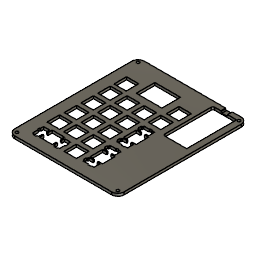
Pad+plate (Autodesk Fusion 360 design; units mm, degrees)
part number: 2026-07-29-07-50-32-719
Autodesk Fusion 360 part; units mm, degrees
(part 1 of 2)
sketch "efc796056b68a6326252bc44c872f28c73b40230_switch" plane through (0, 0, 0) normal (0, 0, 1) x (1, 0, 0)
  line L0 (-14.5057, -35.9059) -> (-14.5057, -40.6078)
  line L1 (-14.5057, -40.6078) -> (-16.0312, -40.6078)
  line L2 (-16.0312, -40.6078) -> (-16.0312, -37.3762)
  line L3 (-16.0312, -37.3762) -> (-22.7808, -37.3762)
  line L4 (-22.7808, -37.3762) -> (-22.7808, -40.6078)
  line L5 (-22.7808, -40.6078) -> (-23.6063, -40.6078)
  line L6 (-23.6063, -40.6078) -> (-23.6063, -43.4066)
  line L7 (-23.6063, -43.4066) -> (-22.7808, -43.4066)
  line L8 (-22.7808, -43.4066) -> (-22.7808, -49.6767)
  line L9 (-22.7808, -49.6767) -> (-21.0555, -49.6767)
  line L10 (-21.0555, -49.6767) -> (-21.0555, -50.8756)
  line L11 (-21.0555, -50.8756) -> (-17.7565, -50.8756)
  line L12 (-17.7565, -50.8756) -> (-17.7565, -49.6767)
  line L13 (-17.7565, -49.6767) -> (-16.0312, -49.6767)
  line L14 (-16.0312, -49.6767) -> (-16.0312, -45.2063)
  line L15 (-16.0312, -45.2063) -> (-14.5057, -45.2063)
  line L16 (-14.5057, -45.2063) -> (-14.5057, -49.9068)
  line L17 (-14.5057, -49.9068) -> (-0.5063, -49.9068)
  line L18 (-0.5063, -49.9068) -> (-0.5063, -45.2063)
  line L19 (-0.5063, -45.2063) -> (1.0192, -45.2063)
  line L20 (1.0192, -45.2063) -> (1.0192, -49.6767)
  line L21 (1.0192, -49.6767) -> (2.7445, -49.6767)
  line L22 (2.7445, -49.6767) -> (2.7445, -50.8756)
  line L23 (2.7445, -50.8756) -> (6.0436, -50.8756)
  line L24 (6.0436, -50.8756) -> (6.0436, -49.6767)
  line L25 (6.0436, -49.6767) -> (7.7689, -49.6767)
  line L26 (7.7689, -49.6767) -> (7.7689, -43.4066)
  line L27 (7.7689, -43.4066) -> (8.5943, -43.4066)
  line L28 (8.5943, -43.4066) -> (8.5943, -40.6078)
  line L29 (8.5943, -40.6078) -> (7.7689, -40.6078)
  line L30 (7.7689, -40.6078) -> (7.7689, -37.3762)
  line L31 (7.7689, -37.3762) -> (1.0192, -37.3762)
  line L32 (1.0192, -37.3762) -> (1.0192, -40.6078)
  line L33 (1.0192, -40.6078) -> (-0.5063, -40.6078)
  line L34 (-0.5063, -40.6078) -> (-0.5063, -35.9059)
  line L35 (-0.5063, -35.9059) -> (-14.5057, -35.9059)
  line L36 (14.0693, -35.9059) -> (28.0686, -35.9059)
  line L37 (28.0686, -35.9059) -> (28.0686, -49.9068)
  line L38 (28.0686, -49.9068) -> (14.0693, -49.9068)
  line L39 (14.0693, -49.9068) -> (14.0693, -35.9059)
  line L40 (39.6196, -17.2817) -> (39.6196, -18.1071)
  line L41 (39.6196, -18.1071) -> (33.3493, -18.1071)
  line L42 (33.3493, -18.1071) -> (33.3493, -19.8325)
  line L43 (33.3493, -19.8325) -> (32.1492, -19.8325)
  line L44 (32.1492, -19.8325) -> (32.1492, -23.1315)
  line L45 (32.1492, -23.1315) -> (33.3493, -23.1315)
  line L46 (33.3493, -23.1315) -> (33.3493, -24.8568)
  line L47 (33.3493, -24.8568) -> (37.8197, -24.8568)
  line L48 (37.8197, -24.8568) -> (37.8197, -26.3823)
  line L49 (37.8197, -26.3823) -> (33.1193, -26.3823)
  line L50 (33.1193, -26.3823) -> (33.1193, -40.3818)
  line L51 (33.1193, -40.3818) -> (37.8197, -40.3818)
  line L52 (37.8197, -40.3818) -> (37.8197, -41.9073)
  line L53 (37.8197, -41.9073) -> (33.3493, -41.9073)
  line L54 (33.3493, -41.9073) -> (33.3493, -43.6326)
  line L55 (33.3493, -43.6326) -> (32.1492, -43.6326)
  line L56 (32.1492, -43.6326) -> (32.1492, -46.9316)
  line L57 (32.1492, -46.9316) -> (33.3493, -46.9316)
  line L58 (33.3493, -46.9316) -> (33.3493, -48.6569)
  line L59 (33.3493, -48.6569) -> (39.6196, -48.6569)
  line L60 (39.6196, -48.6569) -> (39.6196, -49.4824)
  line L61 (39.6196, -49.4824) -> (42.4196, -49.4824)
  line L62 (42.4196, -49.4824) -> (42.4196, -48.6569)
  line L63 (42.4196, -48.6569) -> (45.6496, -48.6569)
  line L64 (45.6496, -48.6569) -> (45.6496, -41.9073)
  line L65 (45.6496, -41.9073) -> (42.4196, -41.9073)
  line L66 (42.4196, -41.9073) -> (42.4196, -40.3818)
  line L67 (42.4196, -40.3818) -> (47.1186, -40.3818)
  line L68 (47.1186, -40.3818) -> (47.1186, -26.3823)
  line L69 (47.1186, -26.3823) -> (42.4196, -26.3823)
  line L70 (42.4196, -26.3823) -> (42.4196, -24.8568)
  line L71 (42.4196, -24.8568) -> (45.6496, -24.8568)
  line L72 (45.6496, -24.8568) -> (45.6496, -18.1071)
  line L73 (45.6496, -18.1071) -> (42.4196, -18.1071)
  line L74 (42.4196, -18.1071) -> (42.4196, -17.2817)
  line L75 (42.4196, -17.2817) -> (39.6196, -17.2817)
  line L76 (-24.0307, -16.8574) -> (-10.0312, -16.8574)
  line L77 (-10.0312, -16.8574) -> (-10.0312, -30.8568)
  line L78 (-10.0312, -30.8568) -> (-24.0307, -30.8568)
  line L79 (-24.0307, -30.8568) -> (-24.0307, -16.8574)
  line L80 (-4.9807, -16.8574) -> (9.0186, -16.8574)
  line L81 (9.0186, -16.8574) -> (9.0186, -30.8568)
  line L82 (9.0186, -30.8568) -> (-4.9807, -30.8568)
  line L83 (-4.9807, -30.8568) -> (-4.9807, -16.8574)
  line L84 (14.0693, -16.8574) -> (28.0686, -16.8574)
  line L85 (28.0686, -16.8574) -> (28.0686, -30.8568)
  line L86 (28.0686, -30.8568) -> (14.0693, -30.8568)
  line L87 (14.0693, -30.8568) -> (14.0693, -16.8574)
  line L88 (-24.0307, 2.1927) -> (-10.0312, 2.1927)
  line L89 (-10.0312, 2.1927) -> (-10.0312, -11.8066)
  line L90 (-10.0312, -11.8066) -> (-24.0307, -11.8066)
  line L91 (-24.0307, -11.8066) -> (-24.0307, 2.1927)
  line L92 (-4.9807, 2.1927) -> (9.0186, 2.1927)
  line L93 (9.0186, 2.1927) -> (9.0186, -11.8066)
  line L94 (9.0186, -11.8066) -> (-4.9807, -11.8066)
  line L95 (-4.9807, -11.8066) -> (-4.9807, 2.1927)
  line L96 (14.0693, 2.1927) -> (28.0686, 2.1927)
  line L97 (28.0686, 2.1927) -> (28.0686, -11.8066)
  line L98 (28.0686, -11.8066) -> (14.0693, -11.8066)
  line L99 (14.0693, -11.8066) -> (14.0693, 2.1927)
  line L100 (39.6196, 20.8183) -> (39.6196, 19.9928)
  line L101 (39.6196, 19.9928) -> (33.3493, 19.9928)
  line L102 (33.3493, 19.9928) -> (33.3493, 18.2691)
  line L103 (33.3493, 18.2691) -> (32.1492, 18.2691)
  line L104 (32.1492, 18.2691) -> (32.1492, 14.9685)
  line L105 (32.1492, 14.9685) -> (33.3493, 14.9685)
  line L106 (33.3493, 14.9685) -> (33.3493, 13.2431)
  line L107 (33.3493, 13.2431) -> (37.8197, 13.2431)
  line L108 (37.8197, 13.2431) -> (37.8197, 11.7177)
  line L109 (37.8197, 11.7177) -> (33.1193, 11.7177)
  line L110 (33.1193, 11.7177) -> (33.1193, -2.2816)
  line L111 (33.1193, -2.2816) -> (37.8197, -2.2816)
  line L112 (37.8197, -2.2816) -> (37.8197, -3.8074)
  line L113 (37.8197, -3.8074) -> (33.3493, -3.8074)
  line L114 (33.3493, -3.8074) -> (33.3493, -5.5325)
  line L115 (33.3493, -5.5325) -> (32.1492, -5.5325)
  line L116 (32.1492, -5.5325) -> (32.1492, -8.8317)
  line L117 (32.1492, -8.8317) -> (33.3493, -8.8317)
  line L118 (33.3493, -8.8317) -> (33.3493, -10.5567)
  line L119 (33.3493, -10.5567) -> (39.6196, -10.5567)
  line L120 (39.6196, -10.5567) -> (39.6196, -11.3822)
  line L121 (39.6196, -11.3822) -> (42.4196, -11.3822)
  line L122 (42.4196, -11.3822) -> (42.4196, -10.5567)
  line L123 (42.4196, -10.5567) -> (45.6496, -10.5567)
  line L124 (45.6496, -10.5567) -> (45.6496, -3.8074)
  line L125 (45.6496, -3.8074) -> (42.4196, -3.8074)
  line L126 (42.4196, -3.8074) -> (42.4196, -2.2816)
  line L127 (42.4196, -2.2816) -> (47.1186, -2.2816)
  line L128 (47.1186, -2.2816) -> (47.1186, 11.7177)
  line L129 (47.1186, 11.7177) -> (42.4196, 11.7177)
  line L130 (42.4196, 11.7177) -> (42.4196, 13.2431)
  line L131 (42.4196, 13.2431) -> (45.6496, 13.2431)
  line L132 (45.6496, 13.2431) -> (45.6496, 19.9928)
  line L133 (45.6496, 19.9928) -> (42.4196, 19.9928)
  line L134 (42.4196, 19.9928) -> (42.4196, 20.8183)
  line L135 (42.4196, 20.8183) -> (39.6196, 20.8183)
  line L136 (-24.0307, 21.2427) -> (-10.0312, 21.2427)
  line L137 (-10.0312, 21.2427) -> (-10.0312, 7.2434)
  line L138 (-10.0312, 7.2434) -> (-24.0307, 7.2434)
  line L139 (-24.0307, 7.2434) -> (-24.0307, 21.2427)
  line L140 (-4.9807, 21.2427) -> (9.0186, 21.2427)
  line L141 (9.0186, 21.2427) -> (9.0186, 7.2434)
  line L142 (9.0186, 7.2434) -> (-4.9807, 7.2434)
  line L143 (-4.9807, 7.2434) -> (-4.9807, 21.2427)
  line L144 (14.0693, 21.2427) -> (28.0686, 21.2427)
  line L145 (28.0686, 21.2427) -> (28.0686, 7.2434)
  line L146 (28.0686, 7.2434) -> (14.0693, 7.2434)
  line L147 (14.0693, 7.2434) -> (14.0693, 21.2427)
  line L148 (-24.0307, 40.2927) -> (-10.0312, 40.2927)
  line L149 (-10.0312, 40.2927) -> (-10.0312, 26.2934)
  line L150 (-10.0312, 26.2934) -> (-24.0307, 26.2934)
  line L151 (-24.0307, 26.2934) -> (-24.0307, 40.2927)
  line L152 (-4.9807, 40.2927) -> (9.0186, 40.2927)
  line L153 (9.0186, 40.2927) -> (9.0186, 26.2934)
  line L154 (9.0186, 26.2934) -> (-4.9807, 26.2934)
  line L155 (-4.9807, 26.2934) -> (-4.9807, 40.2927)
  line L156 (14.0693, 40.2927) -> (28.0686, 40.2927)
  line L157 (28.0686, 40.2927) -> (28.0686, 26.2934)
  line L158 (28.0686, 26.2934) -> (14.0693, 26.2934)
  line L159 (14.0693, 26.2934) -> (14.0693, 40.2927)
  line L160 (33.1193, 40.2927) -> (47.1186, 40.2927)
  line L161 (47.1186, 40.2927) -> (47.1186, 26.2934)
  line L162 (47.1186, 26.2934) -> (33.1193, 26.2934)
  line L163 (33.1193, 26.2934) -> (33.1193, 40.2927)
  line L164 (-24.0307, 59.3426) -> (-10.0312, 59.3426)
  line L165 (-10.0312, 59.3426) -> (-10.0312, 45.3434)
  line L166 (-10.0312, 45.3434) -> (-24.0307, 45.3434)
  line L167 (-24.0307, 45.3434) -> (-24.0307, 59.3426)
  line L168 (33.1193, 59.3426) -> (47.1186, 59.3426)
  line L169 (47.1186, 59.3426) -> (47.1186, 45.3434)
  line L170 (47.1186, 45.3434) -> (33.1193, 45.3434)
  line L171 (33.1193, 45.3434) -> (33.1193, 59.3426)
sketch "Pad_plate _sketch" plane through (0, 0, 0) normal (0, 0, 1) x (1, 0, 0)
  line L0 (-30.0717, -55.8522) -> (79.9283, -55.8522)
  line L1 (79.9283, -55.8522) -> (79.9283, 77.1478)
  line L2 (79.9283, 77.1478) -> (-30.0717, 77.1478)
  line L3 (-30.0717, 77.1478) -> (-30.0717, -55.8522)
  circle A0 centre (74.9283, -50.8522) radius 1.5875
  circle A1 centre (-3.1217, -47.9522) radius 0.3874
  circle A2 centre (25.4533, -47.9522) radius 0.3874
  circle A3 centre (-8.2017, -43.9522) radius 1.9875
  circle A4 centre (20.3733, -43.9522) radius 1.9875
  circle A5 centre (-13.2817, -43.9522) radius 0.8624
  circle A6 centre (-3.1217, -43.9522) radius 0.8624
  circle A7 centre (15.2933, -43.9522) radius 0.8624
  circle A8 centre (25.4533, -43.9522) radius 0.8624
  circle A9 centre (-12.0117, -41.4122) radius 0.7374
  circle A10 centre (16.5633, -41.4122) radius 0.7374
  circle A11 centre (-3.1217, -40.3322) radius 0.3874
  circle A12 centre (25.4533, -40.3322) radius 0.3874
  circle A13 centre (39.4233, -39.5072) radius 0.8624
  circle A14 centre (-5.6617, -38.8722) radius 0.7374
  circle A15 centre (22.9133, -38.8722) radius 0.7374
  circle A16 centre (36.8833, -38.2372) radius 0.7374
  circle A17 centre (44.5033, -38.4272) radius 0.3874
  circle A18 centre (39.4233, -34.4272) radius 1.9875
  circle A19 centre (34.3433, -31.8872) radius 0.7374
  circle A20 centre (44.5033, -30.8072) radius 0.3874
  circle A21 centre (39.4233, -29.3472) radius 0.8624
  circle A22 centre (-12.6467, -28.9022) radius 0.3874
  circle A23 centre (6.4033, -28.9022) radius 0.3874
  circle A24 centre (25.4533, -28.9022) radius 0.3874
  circle A25 centre (-17.7267, -24.9022) radius 1.9875
  circle A26 centre (1.3233, -24.9022) radius 1.9875
  circle A27 centre (20.3733, -24.9022) radius 1.9875
  circle A28 centre (-22.8067, -24.9022) radius 0.8624
  circle A29 centre (-12.6467, -24.9022) radius 0.8624
  circle A30 centre (-3.7567, -24.9022) radius 0.8624
  circle A31 centre (6.4033, -24.9022) radius 0.8624
  circle A32 centre (15.2933, -24.9022) radius 0.8624
  circle A33 centre (25.4533, -24.9022) radius 0.8624
  circle A34 centre (-21.5367, -22.3622) radius 0.7374
  circle A35 centre (-2.4867, -22.3622) radius 0.7374
  circle A36 centre (16.5633, -22.3622) radius 0.7374
  circle A37 centre (-12.6467, -21.2822) radius 0.3874
  circle A38 centre (6.4033, -21.2822) radius 0.3874
  circle A39 centre (25.4533, -21.2822) radius 0.3874
  circle A40 centre (-15.1867, -19.8222) radius 0.7374
  circle A41 centre (3.8633, -19.8222) radius 0.7374
  circle A42 centre (22.9133, -19.8222) radius 0.7374
  circle A43 centre (-12.6467, -9.8522) radius 0.3874
  circle A44 centre (6.4033, -9.8522) radius 0.3874
  circle A45 centre (25.4533, -9.8522) radius 0.3874
  circle A46 centre (-17.7267, -5.8522) radius 1.9875
  circle A47 centre (1.3233, -5.8522) radius 1.9875
  circle A48 centre (20.3733, -5.8522) radius 1.9875
  circle A49 centre (-22.8067, -5.8522) radius 0.8624
  circle A50 centre (-12.6467, -5.8522) radius 0.8624
  circle A51 centre (-3.7567, -5.8522) radius 0.8624
  circle A52 centre (6.4033, -5.8522) radius 0.8624
  circle A53 centre (15.2933, -5.8522) radius 0.8624
  circle A54 centre (25.4533, -5.8522) radius 0.8624
  circle A55 centre (-21.5367, -3.3122) radius 0.7374
  circle A56 centre (-2.4867, -3.3122) radius 0.7374
  circle A57 centre (16.5633, -3.3122) radius 0.7374
  circle A58 centre (-12.6467, -2.2322) radius 0.3874
  circle A59 centre (6.4033, -2.2322) radius 0.3874
  circle A60 centre (25.4533, -2.2322) radius 0.3874
  circle A61 centre (39.4233, -1.4072) radius 0.8624
  circle A62 centre (-15.1867, -0.7722) radius 0.7374
  circle A63 centre (3.8633, -0.7722) radius 0.7374
  circle A64 centre (22.9133, -0.7722) radius 0.7374
  circle A65 centre (36.8833, -0.1372) radius 0.7374
  circle A66 centre (44.5033, -0.3272) radius 0.3874
  circle A67 centre (39.4233, 3.6728) radius 1.9875
  circle A68 centre (34.3433, 6.2128) radius 0.7374
  circle A69 centre (44.5033, 7.2928) radius 0.3874
  circle A70 centre (39.4233, 8.7528) radius 0.8624
  circle A71 centre (-12.6467, 9.1978) radius 0.3874
  circle A72 centre (6.4033, 9.1978) radius 0.3874
  circle A73 centre (25.4533, 9.1978) radius 0.3874
  circle A74 centre (-17.7267, 13.1978) radius 1.9875
  circle A75 centre (1.3233, 13.1978) radius 1.9875
  circle A76 centre (20.3733, 13.1978) radius 1.9875
  circle A77 centre (-22.8067, 13.1978) radius 0.8624
  circle A78 centre (-12.6467, 13.1978) radius 0.8624
  circle A79 centre (-3.7567, 13.1978) radius 0.8624
  circle A80 centre (6.4033, 13.1978) radius 0.8624
  circle A81 centre (15.2933, 13.1978) radius 0.8624
  circle A82 centre (25.4533, 13.1978) radius 0.8624
  circle A83 centre (-21.5367, 15.7378) radius 0.7374
  circle A84 centre (-2.4867, 15.7378) radius 0.7374
  circle A85 centre (16.5633, 15.7378) radius 0.7374
  circle A86 centre (-12.6467, 16.8178) radius 0.3874
  circle A87 centre (6.4033, 16.8178) radius 0.3874
  circle A88 centre (25.4533, 16.8178) radius 0.3874
  circle A89 centre (-15.1867, 18.2778) radius 0.7374
  circle A90 centre (3.8633, 18.2778) radius 0.7374
  circle A91 centre (22.9133, 18.2778) radius 0.7374
  circle A92 centre (57.1483, 27.0478) radius 0.4974
  circle A93 centre (74.9283, 27.0478) radius 0.4974
  circle A94 centre (63.4983, 27.2778) radius 0.4974
  circle A95 centre (66.0383, 27.2778) radius 0.4974
  circle A96 centre (68.5783, 27.2778) radius 0.4974
  circle A97 centre (-12.6467, 28.2478) radius 0.3874
  circle A98 centre (6.4033, 28.2478) radius 0.3874
  circle A99 centre (25.4533, 28.2478) radius 0.3874
  circle A100 centre (44.5033, 28.2478) radius 0.3874
  circle A101 centre (57.1483, 29.5878) radius 0.4974
  circle A102 centre (74.9283, 29.5878) radius 0.4974
  circle A103 centre (-17.7267, 32.2478) radius 1.9875
  circle A104 centre (1.3233, 32.2478) radius 1.9875
  circle A105 centre (20.3733, 32.2478) radius 1.9875
  circle A106 centre (39.4233, 32.2478) radius 1.9875
  circle A107 centre (-22.8067, 32.2478) radius 0.8624
  circle A108 centre (-12.6467, 32.2478) radius 0.8624
  circle A109 centre (-3.7567, 32.2478) radius 0.8624
  circle A110 centre (6.4033, 32.2478) radius 0.8624
  circle A111 centre (15.2933, 32.2478) radius 0.8624
  circle A112 centre (25.4533, 32.2478) radius 0.8624
  circle A113 centre (34.3433, 32.2478) radius 0.8624
  circle A114 centre (44.5033, 32.2478) radius 0.8624
  circle A115 centre (57.1483, 32.1278) radius 0.4974
  circle A116 centre (74.9283, 32.1278) radius 0.4974
  circle A117 centre (-8.5767, 33.7828) radius 0.3874
  circle A118 centre (-21.5367, 34.7878) radius 0.7374
  circle A119 centre (-2.4867, 34.7878) radius 0.7374
  circle A120 centre (16.5633, 34.7878) radius 0.7374
  circle A121 centre (35.6133, 34.7878) radius 0.7374
  circle A122 centre (57.1483, 34.6678) radius 0.4974
  circle A123 centre (74.9283, 34.6678) radius 0.4974
  circle A124 centre (29.4233, 35.7828) radius 0.3874
  circle A125 centre (-12.6467, 35.8678) radius 0.3874
  circle A126 centre (6.4033, 35.8678) radius 0.3874
  circle A127 centre (25.4533, 35.8678) radius 0.3874
  circle A128 centre (44.5033, 35.8678) radius 0.3874
  circle A129 centre (-15.1867, 37.3278) radius 0.7374
  circle A130 centre (3.8633, 37.3278) radius 0.7374
  circle A131 centre (22.9133, 37.3278) radius 0.7374
  circle A132 centre (41.9633, 37.3278) radius 0.7374
  circle A133 centre (57.1483, 37.2078) radius 0.4974
  circle A134 centre (74.9283, 37.2078) radius 0.4974
  circle A135 centre (57.1483, 39.7478) radius 0.4974
  circle A136 centre (74.9283, 39.7478) radius 0.4974
  circle A137 centre (-8.5767, 41.4028) radius 0.3874
  circle A138 centre (57.1483, 42.2878) radius 0.4974
  circle A139 centre (74.9283, 42.2878) radius 0.4974
  circle A140 centre (29.4233, 43.4028) radius 0.3874
  line L4 (-17.927, 45.7303) -> (-19.2264, 45.7303)
  line L5 (-19.9324, 44.7787) -> (-19.8771, 44.6451)
  arc A141 (-19.2264, 45.7303) -> (-19.9324, 44.7787) centre (-19.2266, 44.9928) ccw
  arc A142 (-17.927, 44.2553) -> (-17.927, 45.7303) centre (-17.9268, 44.9928) ccw
  arc A143 (-19.8771, 44.6451) -> (-19.2264, 44.2553) centre (-19.2265, 44.9929) ccw
  line L6 (-19.2264, 44.2553) -> (-17.927, 44.2553)
  circle A144 centre (57.1483, 44.8278) radius 0.4974
  circle A145 centre (74.9283, 44.8278) radius 0.4974
  line L7 (41.073, 46.2303) -> (39.7736, 46.2303)
  arc A146 (39.7736, 46.2303) -> (39.0676, 45.2787) centre (39.7734, 45.4928) ccw
  arc A147 (39.1229, 45.1451) -> (39.7736, 44.7553) centre (39.7735, 45.4929) ccw
  line L8 (39.0676, 45.2787) -> (39.1229, 45.1451)
  arc A148 (41.073, 44.7553) -> (41.073, 46.2303) centre (41.0732, 45.4928) ccw
  line L9 (39.7736, 44.7553) -> (41.073, 44.7553)
  circle A149 centre (57.1483, 47.3678) radius 0.4974
  circle A150 centre (74.9283, 47.3678) radius 0.4974
  circle A151 centre (-26.0767, 48.0928) radius 0.4874
  circle A152 centre (-11.5767, 48.0928) radius 0.4874
  circle A153 centre (32.9233, 48.5928) radius 0.4874
  circle A154 centre (47.4233, 48.5928) radius 0.4874
  circle A155 centre (0.4238, 49.6478) radius 1.0875
  circle A156 centre (7.1183, 49.1478) radius 0.4874
  circle A157 centre (9.6583, 49.1478) radius 0.4874
  circle A158 centre (12.1983, 49.1478) radius 0.4874
  circle A159 centre (14.7383, 49.1478) radius 0.4874
  circle A160 centre (57.1483, 49.9078) radius 0.4974
  circle A161 centre (74.9283, 49.9078) radius 0.4974
  circle A162 centre (-18.5767, 50.5928) radius 1.0374
  line L10 (-23.3764, 49.8053) -> (-22.777, 49.8053)
  line L11 (-24.1302, 50.3642) -> (-24.0712, 50.2216)
  arc A163 (-22.777, 49.8053) -> (-22.777, 51.3803) centre (-22.7768, 50.5928) ccw
  arc A164 (-23.3764, 51.3803) -> (-24.1302, 50.3642) centre (-23.3766, 50.5928) ccw
  line L12 (-22.777, 51.3803) -> (-23.3764, 51.3803)
  arc A165 (-24.0712, 50.2216) -> (-23.3764, 49.8053) centre (-23.3765, 50.5929) ccw
  circle A166 centre (40.4233, 51.0928) radius 1.0374
  circle A167 centre (-26.0767, 50.5928) radius 0.4874
  line L13 (34.8698, 50.8642) -> (34.9288, 50.7216)
  arc A168 (35.6236, 51.8803) -> (34.8698, 50.8642) centre (35.6234, 51.0928) ccw
  line L14 (35.6236, 50.3053) -> (36.223, 50.3053)
  line L15 (36.223, 51.8803) -> (35.6236, 51.8803)
  arc A169 (34.9288, 50.7216) -> (35.6236, 50.3053) centre (35.6235, 51.0929) ccw
  arc A170 (36.223, 50.3053) -> (36.223, 51.8803) centre (36.2232, 51.0928) ccw
  circle A171 centre (32.9233, 51.0928) radius 0.4874
  circle A172 centre (57.1483, 52.4478) radius 0.4974
  circle A173 centre (74.9283, 52.4478) radius 0.4974
  circle A174 centre (-26.0767, 53.0928) radius 0.4874
  circle A175 centre (-11.5767, 53.0928) radius 0.4874
  circle A176 centre (32.9233, 53.5928) radius 0.4874
  circle A177 centre (47.4233, 53.5928) radius 0.4874
  circle A178 centre (57.1483, 54.9878) radius 0.4974
  circle A179 centre (74.9283, 54.9878) radius 0.4974
  arc A180 (-19.2264, 56.9303) -> (-19.9324, 55.9787) centre (-19.2266, 56.1928) ccw
  arc A181 (-17.927, 55.4553) -> (-17.927, 56.9303) centre (-17.9268, 56.1928) ccw
  line L16 (-19.2264, 55.4553) -> (-17.927, 55.4553)
  line L17 (-19.9324, 55.9787) -> (-19.8771, 55.8451)
  arc A182 (-19.8771, 55.8451) -> (-19.2264, 55.4553) centre (-19.2265, 56.1929) ccw
  line L18 (-17.927, 56.9303) -> (-19.2264, 56.9303)
  line L19 (39.0676, 56.4787) -> (39.1229, 56.3451)
  arc A183 (39.7736, 57.4303) -> (39.0676, 56.4787) centre (39.7734, 56.6928) ccw
  line L20 (41.073, 57.4303) -> (39.7736, 57.4303)
  arc A184 (41.073, 55.9553) -> (41.073, 57.4303) centre (41.0732, 56.6928) ccw
  arc A185 (39.1229, 56.3451) -> (39.7736, 55.9553) centre (39.7735, 56.6929) ccw
  line L21 (39.7736, 55.9553) -> (41.073, 55.9553)
  circle A186 centre (57.1483, 57.5278) radius 0.4974
  circle A187 centre (74.9283, 57.5278) radius 0.4974
  circle A188 centre (57.1483, 60.0678) radius 0.4974
  circle A189 centre (74.9283, 60.0678) radius 0.4974
  circle A190 centre (57.1483, 62.6078) radius 0.4974
  circle A191 centre (74.9283, 62.6078) radius 0.4974
  circle A192 centre (57.1483, 65.1478) radius 0.4974
  circle A193 centre (74.9283, 65.1478) radius 0.4974
  circle A194 centre (57.1483, 67.6878) radius 0.4974
  circle A195 centre (74.9283, 67.6878) radius 0.4974
  circle A196 centre (-26.0717, 70.1478) radius 1.5875
  circle A197 centre (57.1483, 70.2278) radius 0.4974
  circle A198 centre (74.9283, 70.2278) radius 0.4974
  circle A199 centre (0.4238, 72.6478) radius 1.0875
  circle A200 centre (21.4283, 72.6478) radius 1.0875
  circle A201 centre (57.1483, 72.7678) radius 0.4974
  circle A202 centre (74.9283, 72.7678) radius 0.4974
  circle A203 centre (57.1483, 75.3078) radius 0.4974
  circle A204 centre (74.9283, 75.3078) radius 0.4974
  line L22 (74.9383, 35.4678) -> (76.5383, 35.4678)
  line L23 (65.2383, 25.6778) -> (65.2383, 27.8778)
  line L24 (76.5383, 46.5678) -> (74.9383, 46.5678)
  arc A205 (66.6383, 28.0778) -> (66.8383, 27.8778) centre (66.6383, 27.8778) cw
  line L25 (74.1383, 31.5278) -> (74.1383, 32.7278)
  line L26 (76.5383, 28.7878) -> (74.9383, 28.7878)
  arc A206 (67.7783, 27.2778) -> (69.3783, 27.2778) centre (68.5783, 27.2778) cw
  line L27 (74.9383, 50.7078) -> (76.5383, 50.7078)
  line L28 (76.5383, 26.2478) -> (74.9383, 26.2478)
  arc A207 (74.9383, 28.7878) -> (74.9383, 30.3878) centre (74.9383, 29.5878) cw
  line L29 (74.9383, 48.1678) -> (76.5383, 48.1678)
  arc A208 (74.9383, 46.5678) -> (74.9383, 48.1678) centre (74.9383, 47.3678) cw
  line L30 (76.5383, 49.1078) -> (74.9383, 49.1078)
  line L31 (74.9383, 40.5478) -> (76.5383, 40.5478)
  arc A209 (74.3383, 44.0278) -> (74.1383, 44.2278) centre (74.3383, 44.2278) cw
  line L32 (76.5383, 25.6778) -> (76.5383, 26.2478)
  line L33 (76.5383, 48.1678) -> (76.5383, 49.1078)
  line L34 (69.3783, 27.2778) -> (69.3783, 25.6778)
  line L35 (76.5383, 30.3878) -> (76.5383, 31.3278)
  arc A210 (74.9383, 38.9478) -> (74.9383, 40.5478) centre (74.9383, 39.7478) cw
  line L36 (74.9383, 27.8478) -> (76.5383, 27.8478)
  line L37 (76.5383, 31.3278) -> (74.3383, 31.3278)
  arc A211 (74.9383, 26.2478) -> (74.9383, 27.8478) centre (74.9383, 27.0478) cw
  line L38 (76.5383, 36.4078) -> (74.9383, 36.4078)
  line L39 (74.3383, 32.9278) -> (76.5383, 32.9278)
  line L40 (76.5383, 33.8678) -> (74.9383, 33.8678)
  arc A212 (65.2383, 27.8778) -> (65.4383, 28.0778) centre (65.4383, 27.8778) cw
  line L41 (69.3783, 25.6778) -> (76.5383, 25.6778)
  line L42 (76.5383, 44.0278) -> (74.3383, 44.0278)
  arc A213 (74.9383, 36.4078) -> (74.9383, 38.0078) centre (74.9383, 37.2078) cw
  line L43 (66.8383, 25.6778) -> (67.7783, 25.6778)
  line L44 (76.5383, 43.0878) -> (76.5383, 44.0278)
  line L45 (76.5383, 40.5478) -> (76.5383, 41.4878)
  line L46 (74.9383, 38.0078) -> (76.5383, 38.0078)
  arc A214 (74.9383, 33.8678) -> (74.9383, 35.4678) centre (74.9383, 34.6678) cw
  arc A215 (74.9383, 49.1078) -> (74.9383, 50.7078) centre (74.9383, 49.9078) cw
  line L47 (74.3383, 45.6278) -> (76.5383, 45.6278)
  arc A216 (74.3383, 31.3278) -> (74.1383, 31.5278) centre (74.3383, 31.5278) cw
  line L48 (74.9383, 55.7878) -> (76.5383, 55.7878)
  line L49 (76.5383, 38.9478) -> (74.9383, 38.9478)
  line L50 (74.1383, 69.6278) -> (74.1383, 70.8278)
  arc A217 (74.9383, 41.4878) -> (74.9383, 43.0878) centre (74.9383, 42.2878) cw
  line L51 (74.1383, 44.2278) -> (74.1383, 45.4278)
  line L52 (65.4383, 28.0778) -> (66.6383, 28.0778)
  line L53 (76.5383, 61.8078) -> (74.9383, 61.8078)
  arc A218 (74.1383, 32.7278) -> (74.3383, 32.9278) centre (74.3383, 32.7278) cw
  line L54 (76.5383, 35.4678) -> (76.5383, 36.4078)
  line L55 (66.8383, 27.8778) -> (66.8383, 25.6778)
  line L56 (76.5383, 32.9278) -> (76.5383, 33.8678)
  line L57 (76.5383, 27.8478) -> (76.5383, 28.7878)
  line L58 (74.9383, 30.3878) -> (76.5383, 30.3878)
  line L59 (76.5383, 38.0078) -> (76.5383, 38.9478)
  line L60 (74.9383, 43.0878) -> (76.5383, 43.0878)
  line L61 (76.5383, 41.4878) -> (74.9383, 41.4878)
  arc A219 (74.1383, 45.4278) -> (74.3383, 45.6278) centre (74.3383, 45.4278) cw
  line L62 (76.5383, 45.6278) -> (76.5383, 46.5678)
  line L63 (57.9383, 70.8278) -> (57.9383, 69.6278)
  line L64 (67.7783, 25.6778) -> (67.7783, 27.2778)
  line L65 (57.1383, 66.8878) -> (55.5383, 66.8878)
  line L66 (76.5383, 66.8878) -> (74.9383, 66.8878)
  line L67 (57.7383, 69.4278) -> (55.5383, 69.4278)
  line L68 (76.5383, 64.3478) -> (74.9383, 64.3478)
  arc A220 (74.9383, 64.3478) -> (74.9383, 65.9478) centre (74.9383, 65.1478) cw
  arc A221 (74.1383, 58.1278) -> (74.3383, 58.3278) centre (74.3383, 58.1278) cw
  line L69 (55.5383, 76.6778) -> (55.5383, 76.1078)
  line L70 (74.1383, 56.9278) -> (74.1383, 58.1278)
  arc A222 (57.1383, 68.4878) -> (57.1383, 66.8878) centre (57.1383, 67.6878) cw
  line L71 (55.5383, 71.0278) -> (57.7383, 71.0278)
  line L72 (76.5383, 71.0278) -> (76.5383, 71.9678)
  line L73 (74.9383, 68.4878) -> (76.5383, 68.4878)
  line L74 (55.5383, 74.5078) -> (55.5383, 73.5678)
  line L75 (74.9383, 60.8678) -> (76.5383, 60.8678)
  line L76 (76.5383, 55.7878) -> (76.5383, 56.7278)
  line L77 (74.9383, 76.1078) -> (76.5383, 76.1078)
  line L78 (57.1383, 71.9678) -> (55.5383, 71.9678)
  arc A223 (74.9383, 54.1878) -> (74.9383, 55.7878) centre (74.9383, 54.9878) cw
  line L79 (76.5383, 59.2678) -> (74.9383, 59.2678)
  arc A224 (57.9383, 69.6278) -> (57.7383, 69.4278) centre (57.7383, 69.6278) cw
  arc A225 (74.9383, 71.9678) -> (74.9383, 73.5678) centre (74.9383, 72.7678) cw
  arc A226 (74.9383, 51.6478) -> (74.9383, 53.2478) centre (74.9383, 52.4478) cw
  line L80 (76.5383, 58.3278) -> (76.5383, 59.2678)
  line L81 (76.5383, 68.4878) -> (76.5383, 69.4278)
  arc A227 (57.1383, 73.5678) -> (57.1383, 71.9678) centre (57.1383, 72.7678) cw
  line L82 (55.5383, 71.9678) -> (55.5383, 71.0278)
  arc A228 (57.7383, 71.0278) -> (57.9383, 70.8278) centre (57.7383, 70.8278) cw
  line L83 (57.1383, 64.3478) -> (55.5383, 64.3478)
  line L84 (55.5383, 58.3278) -> (57.7383, 58.3278)
  line L85 (55.5383, 76.1078) -> (57.1383, 76.1078)
  line L86 (55.5383, 69.4278) -> (55.5383, 68.4878)
  line L87 (76.5383, 63.4078) -> (76.5383, 64.3478)
  arc A229 (74.9383, 74.5078) -> (74.9383, 76.1078) centre (74.9383, 75.3078) cw
  line L88 (74.3383, 71.0278) -> (76.5383, 71.0278)
  line L89 (76.5383, 76.6778) -> (55.5383, 76.6778)
  line L90 (57.1383, 74.5078) -> (55.5383, 74.5078)
  line L91 (74.9383, 53.2478) -> (76.5383, 53.2478)
  arc A230 (74.9383, 61.8078) -> (74.9383, 63.4078) centre (74.9383, 62.6078) cw
  line L92 (74.3383, 58.3278) -> (76.5383, 58.3278)
  arc A231 (74.9383, 66.8878) -> (74.9383, 68.4878) centre (74.9383, 67.6878) cw
  arc A232 (74.9383, 59.2678) -> (74.9383, 60.8678) centre (74.9383, 60.0678) cw
  line L93 (76.5383, 65.9478) -> (76.5383, 66.8878)
  line L94 (76.5383, 71.9678) -> (74.9383, 71.9678)
  line L95 (76.5383, 60.8678) -> (76.5383, 61.8078)
  arc A233 (74.3383, 56.7278) -> (74.1383, 56.9278) centre (74.3383, 56.9278) cw
  line L96 (76.5383, 69.4278) -> (74.3383, 69.4278)
  line L97 (74.9383, 63.4078) -> (76.5383, 63.4078)
  arc A234 (57.1383, 76.1078) -> (57.1383, 74.5078) centre (57.1383, 75.3078) cw
  line L98 (74.9383, 73.5678) -> (76.5383, 73.5678)
  line L99 (76.5383, 51.6478) -> (74.9383, 51.6478)
  line L100 (76.5383, 54.1878) -> (74.9383, 54.1878)
  line L101 (76.5383, 74.5078) -> (74.9383, 74.5078)
  line L102 (76.5383, 56.7278) -> (74.3383, 56.7278)
  arc A235 (74.1383, 70.8278) -> (74.3383, 71.0278) centre (74.3383, 70.8278) cw
  arc A236 (74.3383, 69.4278) -> (74.1383, 69.6278) centre (74.3383, 69.6278) cw
  line L103 (76.5383, 50.7078) -> (76.5383, 51.6478)
  line L104 (76.5383, 53.2478) -> (76.5383, 54.1878)
  line L105 (55.5383, 73.5678) -> (57.1383, 73.5678)
  line L106 (76.5383, 73.5678) -> (76.5383, 74.5078)
  line L107 (76.5383, 76.1078) -> (76.5383, 76.6778)
  line L108 (74.9383, 65.9478) -> (76.5383, 65.9478)
  line L109 (55.5383, 68.4878) -> (57.1383, 68.4878)
  line L110 (55.5383, 38.0078) -> (57.1383, 38.0078)
  line L111 (55.5383, 66.8878) -> (55.5383, 65.9478)
  line L112 (55.5383, 55.7878) -> (57.1383, 55.7878)
  line L113 (55.5383, 60.8678) -> (57.1383, 60.8678)
  arc A237 (57.1383, 55.7878) -> (57.1383, 54.1878) centre (57.1383, 54.9878) cw
  arc A238 (57.7383, 58.3278) -> (57.9383, 58.1278) centre (57.7383, 58.1278) cw
  line L114 (57.9383, 32.7278) -> (57.9383, 31.5278)
  arc A239 (57.1383, 48.1678) -> (57.1383, 46.5678) centre (57.1383, 47.3678) cw
  line L115 (57.7383, 44.0278) -> (55.5383, 44.0278)
  line L116 (57.7383, 31.3278) -> (55.5383, 31.3278)
  line L117 (55.5383, 31.3278) -> (55.5383, 30.3878)
  line L118 (55.5383, 38.9478) -> (55.5383, 38.0078)
  line L119 (55.5383, 35.4678) -> (57.1383, 35.4678)
  line L120 (57.1383, 54.1878) -> (55.5383, 54.1878)
  line L121 (57.9383, 58.1278) -> (57.9383, 56.9278)
  line L122 (57.1383, 49.1078) -> (55.5383, 49.1078)
  line L123 (55.5383, 65.9478) -> (57.1383, 65.9478)
  line L124 (55.5383, 53.2478) -> (57.1383, 53.2478)
  arc A240 (57.1383, 53.2478) -> (57.1383, 51.6478) centre (57.1383, 52.4478) cw
  arc A241 (57.1383, 60.8678) -> (57.1383, 59.2678) centre (57.1383, 60.0678) cw
  line L125 (57.9383, 45.4278) -> (57.9383, 44.2278)
  arc A242 (57.7383, 32.9278) -> (57.9383, 32.7278) centre (57.7383, 32.7278) cw
  line L126 (55.5383, 61.8078) -> (55.5383, 60.8678)
  line L127 (57.1383, 46.5678) -> (55.5383, 46.5678)
  line L128 (57.1383, 41.4878) -> (55.5383, 41.4878)
  line L129 (55.5383, 46.5678) -> (55.5383, 45.6278)
  arc A243 (57.1383, 38.0078) -> (57.1383, 36.4078) centre (57.1383, 37.2078) cw
  line L130 (57.1383, 61.8078) -> (55.5383, 61.8078)
  line L131 (57.1383, 51.6478) -> (55.5383, 51.6478)
  arc A244 (57.1383, 50.7078) -> (57.1383, 49.1078) centre (57.1383, 49.9078) cw
  line L132 (55.5383, 56.7278) -> (55.5383, 55.7878)
  line L133 (55.5383, 63.4078) -> (57.1383, 63.4078)
  line L134 (57.1383, 59.2678) -> (55.5383, 59.2678)
  line L135 (55.5383, 50.7078) -> (57.1383, 50.7078)
  line L136 (55.5383, 30.3878) -> (57.1383, 30.3878)
  line L137 (57.7383, 56.7278) -> (55.5383, 56.7278)
  arc A245 (57.1383, 63.4078) -> (57.1383, 61.8078) centre (57.1383, 62.6078) cw
  arc A246 (57.9383, 31.5278) -> (57.7383, 31.3278) centre (57.7383, 31.5278) cw
  line L138 (55.5383, 54.1878) -> (55.5383, 53.2478)
  line L139 (55.5383, 49.1078) -> (55.5383, 48.1678)
  arc A247 (57.7383, 45.6278) -> (57.9383, 45.4278) centre (57.7383, 45.4278) cw
  line L140 (55.5383, 41.4878) -> (55.5383, 40.5478)
  arc A248 (57.1383, 65.9478) -> (57.1383, 64.3478) centre (57.1383, 65.1478) cw
  line L141 (57.1383, 38.9478) -> (55.5383, 38.9478)
  line L142 (55.5383, 51.6478) -> (55.5383, 50.7078)
  line L143 (55.5383, 64.3478) -> (55.5383, 63.4078)
  line L144 (55.5383, 40.5478) -> (57.1383, 40.5478)
  arc A249 (57.9383, 44.2278) -> (57.7383, 44.0278) centre (57.7383, 44.2278) cw
  arc A250 (57.1383, 43.0878) -> (57.1383, 41.4878) centre (57.1383, 42.2878) cw
  line L145 (55.5383, 32.9278) -> (57.7383, 32.9278)
  arc A251 (62.6983, 27.2778) -> (64.2983, 27.2778) centre (63.4983, 27.2778) cw
  line L146 (55.5383, 59.2678) -> (55.5383, 58.3278)
  line L147 (55.5383, 48.1678) -> (57.1383, 48.1678)
  line L148 (55.5383, 26.2478) -> (55.5383, 25.6778)
  line L149 (55.5383, 45.6278) -> (57.7383, 45.6278)
  line L150 (57.1383, 36.4078) -> (55.5383, 36.4078)
  line L151 (57.1383, 33.8678) -> (55.5383, 33.8678)
  line L152 (55.5383, 44.0278) -> (55.5383, 43.0878)
  arc A252 (57.1383, 35.4678) -> (57.1383, 33.8678) centre (57.1383, 34.6678) cw
  line L153 (55.5383, 28.7878) -> (55.5383, 27.8478)
  arc A253 (57.1383, 27.8478) -> (57.1383, 26.2478) centre (57.1383, 27.0478) cw
  line L154 (55.5383, 25.6778) -> (62.6983, 25.6778)
  line L155 (62.6983, 25.6778) -> (62.6983, 27.2778)
  line L156 (64.2983, 25.6778) -> (65.2383, 25.6778)
  line L157 (55.5383, 27.8478) -> (57.1383, 27.8478)
  line L158 (55.5383, 33.8678) -> (55.5383, 32.9278)
  arc A254 (57.9383, 56.9278) -> (57.7383, 56.7278) centre (57.7383, 56.9278) cw
  line L159 (64.2983, 27.2778) -> (64.2983, 25.6778)
  line L160 (55.5383, 43.0878) -> (57.1383, 43.0878)
  line L161 (57.1383, 26.2478) -> (55.5383, 26.2478)
  arc A255 (57.1383, 40.5478) -> (57.1383, 38.9478) centre (57.1383, 39.7478) cw
  line L162 (55.5383, 36.4078) -> (55.5383, 35.4678)
  arc A256 (57.1383, 30.3878) -> (57.1383, 28.7878) centre (57.1383, 29.5878) cw
  line L163 (57.1383, 28.7878) -> (55.5383, 28.7878)
  circle A257 centre (71.7383, 74.6778) radius 1.9
  circle A258 centre (60.3383, 74.6778) radius 1.9
  circle A259 centre (71.7383, 27.6778) radius 1.9
  circle A260 centre (60.3383, 27.6778) radius 1.9
  line L164 (0.5583, 64.5578) -> (0.5583, 54.6978)
  line L165 (0.5583, 54.6978) -> (21.2983, 54.6978)
  line L166 (21.2983, 54.6978) -> (21.2983, 64.5578)
  line L167 (21.2983, 64.5578) -> (0.5583, 64.5578)
  line L168 (46.4733, 45.5428) -> (46.4733, 56.6428)
  line L169 (41.5733, 45.1428) -> (46.2733, 45.1428)
  arc A261 (46.2733, 45.1428) -> (46.4733, 45.5428) centre (45.9733, 45.5428) ccw
  arc A262 (41.5733, 54.9761) -> (41.5733, 47.2095) centre (40.4233, 51.0928) cw
  arc A263 (46.4733, 56.6428) -> (46.2733, 57.0428) centre (45.9733, 56.6428) ccw
  line L170 (41.5733, 47.2095) -> (41.5733, 45.1428)
  line L171 (41.5733, 57.0428) -> (41.5733, 54.9761)
  arc A264 (34.3733, 45.5428) -> (34.5733, 45.1428) centre (34.8733, 45.5428) ccw
  arc A265 (39.2733, 47.2095) -> (39.2733, 54.9761) centre (40.4233, 51.0928) cw
  line L172 (39.2733, 57.0428) -> (34.5733, 57.0428)
  line L173 (34.5733, 45.1428) -> (39.2733, 45.1428)
  arc A266 (34.5733, 57.0428) -> (34.3733, 56.6428) centre (34.8733, 56.6428) ccw
  line L174 (34.3733, 56.6428) -> (34.3733, 45.5428)
  line L175 (39.2733, 54.9761) -> (39.2733, 57.0428)
  line L176 (39.2733, 45.1428) -> (39.2733, 47.2095)
  line L177 (-17.4267, 56.5428) -> (-17.4267, 54.4761)
  line L178 (-12.5267, 45.0428) -> (-12.5267, 56.1428)
  line L179 (-17.4267, 46.7095) -> (-17.4267, 44.6428)
  line L180 (-12.7267, 56.5428) -> (-17.4267, 56.5428)
  arc A267 (-17.4267, 54.4761) -> (-17.4267, 46.7095) centre (-18.5767, 50.5928) cw
  line L181 (-17.4267, 44.6428) -> (-12.7267, 44.6428)
  arc A268 (-12.7267, 44.6428) -> (-12.5267, 45.0428) centre (-13.0267, 45.0428) ccw
  arc A269 (-24.6267, 45.0428) -> (-24.4267, 44.6428) centre (-24.1267, 45.0428) ccw
  line L182 (-24.4267, 44.6428) -> (-19.7267, 44.6428)
  line L183 (-19.7267, 54.4761) -> (-19.7267, 56.5428)
  line L184 (-19.7267, 44.6428) -> (-19.7267, 46.7095)
  arc A270 (-19.7267, 46.7095) -> (-19.7267, 54.4761) centre (-18.5767, 50.5928) cw
  line L185 (-24.6267, 56.1428) -> (-24.6267, 45.0428)
  arc A271 (-24.4267, 56.5428) -> (-24.6267, 56.1428) centre (-24.1267, 56.1428) ccw
  line L186 (-19.7267, 56.5428) -> (-24.4267, 56.5428)
  line L187 (37.5162, 31.6907) -> (38.9662, 31.6907)
  line L188 (39.8662, 31.6907) -> (41.3162, 31.6907)
  line L189 (38.9662, 30.3407) -> (39.8662, 30.3407)
  line L190 (41.3162, 31.6907) -> (41.3162, 32.7907)
  line L191 (39.8662, 34.1407) -> (38.9662, 34.1407)
  line L192 (41.3162, 32.7907) -> (39.8662, 32.7907)
  line L193 (38.9662, 32.7907) -> (37.5162, 32.7907)
  line L194 (38.9662, 34.1407) -> (38.9662, 32.7907)
  line L195 (39.8662, 32.7907) -> (39.8662, 34.1407)
  line L196 (39.8662, 30.3407) -> (39.8662, 31.6907)
  line L197 (37.5162, 32.7907) -> (37.5162, 31.6907)
  line L198 (38.9662, 31.6907) -> (38.9662, 30.3407)
  line L199 (22.2662, 31.6907) -> (22.2662, 32.7907)
  line L200 (20.8162, 30.3407) -> (20.8162, 31.6907)
  line L201 (20.8162, 31.6907) -> (22.2662, 31.6907)
  line L202 (19.9162, 30.3407) -> (20.8162, 30.3407)
  line L203 (20.8162, 34.1407) -> (19.9162, 34.1407)
  line L204 (20.8162, 32.7907) -> (20.8162, 34.1407)
  line L205 (18.4662, 31.6907) -> (19.9162, 31.6907)
  line L206 (19.9162, 32.7907) -> (18.4662, 32.7907)
  line L207 (19.9162, 31.6907) -> (19.9162, 30.3407)
  line L208 (18.4662, 32.7907) -> (18.4662, 31.6907)
  line L209 (22.2662, 32.7907) -> (20.8162, 32.7907)
  line L210 (19.9162, 34.1407) -> (19.9162, 32.7907)
  line L211 (41.3304, 3.2157) -> (41.3304, 4.1157)
  line L212 (39.9804, 5.5657) -> (38.8804, 5.5657)
  line L213 (39.9804, 1.7657) -> (39.9804, 3.2157)
  line L214 (38.8804, 1.7657) -> (39.9804, 1.7657)
  line L215 (37.5304, 3.2157) -> (38.8804, 3.2157)
  line L216 (38.8804, 3.2157) -> (38.8804, 1.7657)
  line L217 (38.8804, 5.5657) -> (38.8804, 4.1157)
  line L218 (39.9804, 3.2157) -> (41.3304, 3.2157)
  line L219 (37.5304, 4.1157) -> (37.5304, 3.2157)
  line L220 (41.3304, 4.1157) -> (39.9804, 4.1157)
  line L221 (39.9804, 4.1157) -> (39.9804, 5.5657)
  line L222 (38.8804, 4.1157) -> (37.5304, 4.1157)
  line L223 (19.9162, -6.4093) -> (19.9162, -7.7593)
  line L224 (20.8162, -6.4093) -> (22.2662, -6.4093)
  line L225 (19.9162, -5.3093) -> (18.4662, -5.3093)
  line L226 (20.8162, -7.7593) -> (20.8162, -6.4093)
  line L227 (19.9162, -3.9593) -> (19.9162, -5.3093)
  line L228 (22.2662, -5.3093) -> (20.8162, -5.3093)
  line L229 (20.8162, -3.9593) -> (19.9162, -3.9593)
  line L230 (18.4662, -5.3093) -> (18.4662, -6.4093)
  line L231 (19.9162, -7.7593) -> (20.8162, -7.7593)
  line L232 (22.2662, -6.4093) -> (22.2662, -5.3093)
  line L233 (20.8162, -5.3093) -> (20.8162, -3.9593)
  line L234 (18.4662, -6.4093) -> (19.9162, -6.4093)
  line L235 (-30.0717, 77.1478) -> (79.9283, 77.1478)
  line L236 (-30.0717, -55.8522) -> (-30.0717, 77.1478)
  line L237 (79.9283, 77.1478) -> (79.9283, -55.8522)
  line L238 (79.9283, -55.8522) -> (-30.0717, -55.8522)
  line L239 (-17.2838, 11.2907) -> (-17.2838, 12.6407)
  line L240 (-19.6338, 12.6407) -> (-18.1838, 12.6407)
  line L241 (-18.1838, 15.0907) -> (-18.1838, 13.7407)
  line L242 (-18.1838, 11.2907) -> (-17.2838, 11.2907)
  line L243 (-17.2838, 13.7407) -> (-17.2838, 15.0907)
  line L244 (-18.1838, 12.6407) -> (-18.1838, 11.2907)
  line L245 (-15.8338, 13.7407) -> (-17.2838, 13.7407)
  line L246 (-19.6338, 13.7407) -> (-19.6338, 12.6407)
  line L247 (-17.2838, 12.6407) -> (-15.8338, 12.6407)
  line L248 (-18.1838, 13.7407) -> (-19.6338, 13.7407)
  line L249 (-15.8338, 12.6407) -> (-15.8338, 13.7407)
  line L250 (-17.2838, 15.0907) -> (-18.1838, 15.0907)
  line L251 (-12.9338, -0.0171) -> (-22.5338, -0.0171)
  line L252 (-21.8838, -12.1393) -> (-21.8838, -12.2255)
  ellipse E0 centre (-22.0838, -12.3393) end of major axis (-22.261, -12.5165) minor radius 0.1313 (-22.0838, -12.5037) -> (-21.8838, -12.2255) ccw
  line L253 (-22.0838, -12.5037) -> (-13.3838, -12.5037)
  ellipse E1 centre (-13.3838, -12.3393) end of major axis (-13.2066, -12.5165) minor radius 0.1313 (-13.5838, -12.2255) -> (-13.3838, -12.5037) ccw
  line L254 (-13.5838, -12.2255) -> (-13.5838, -12.1393)
  line L255 (-13.5838, -12.1393) -> (-21.8838, -12.1393)
  line L256 (-12.9338, -19.0671) -> (-22.5338, -19.0671)
  line L257 (-13.3838, -31.5537) -> (-22.0838, -31.5537)
  line L258 (5.6162, -19.9005) -> (-2.9838, -19.9005)
  line L259 (5.6662, -31.5537) -> (-3.0338, -31.5537)
  line L260 (-6.3088, -43.4093) -> (-7.7588, -43.4093)
  line L261 (-7.7588, -44.5093) -> (-6.3088, -44.5093)
  line L262 (-7.7588, -42.0593) -> (-8.6588, -42.0593)
  line L263 (-8.6588, -42.0593) -> (-8.6588, -43.4093)
  line L264 (-8.6588, -44.5093) -> (-8.6588, -45.8593)
  line L265 (-7.7588, -43.4093) -> (-7.7588, -42.0593)
  line L266 (-6.3088, -44.5093) -> (-6.3088, -43.4093)
  line L267 (-10.1088, -44.5093) -> (-8.6588, -44.5093)
  line L268 (-10.1088, -43.4093) -> (-10.1088, -44.5093)
  line L269 (-7.7588, -45.8593) -> (-7.7588, -44.5093)
  line L270 (-8.6588, -43.4093) -> (-10.1088, -43.4093)
  line L271 (-8.6588, -45.8593) -> (-7.7588, -45.8593)
  line L272 (19.9162, -43.4093) -> (18.4662, -43.4093)
  line L273 (19.9162, -44.5093) -> (19.9162, -45.8593)
  line L274 (19.9162, -42.0593) -> (19.9162, -43.4093)
  line L275 (20.8162, -45.8593) -> (20.8162, -44.5093)
  line L276 (22.2662, -44.5093) -> (22.2662, -43.4093)
  line L277 (18.4662, -44.5093) -> (19.9162, -44.5093)
  line L278 (22.2662, -43.4093) -> (20.8162, -43.4093)
  line L279 (20.8162, -43.4093) -> (20.8162, -42.0593)
  line L280 (20.8162, -42.0593) -> (19.9162, -42.0593)
  line L281 (20.8162, -44.5093) -> (22.2662, -44.5093)
  line L282 (18.4662, -43.4093) -> (18.4662, -44.5093)
  line L283 (19.9162, -45.8593) -> (20.8162, -45.8593)
  line L284 (38.8804, -34.8843) -> (38.8804, -36.3343)
  line L285 (39.9804, -32.5343) -> (38.8804, -32.5343)
  line L286 (39.9804, -34.8843) -> (41.3304, -34.8843)
  line L287 (39.9804, -36.3343) -> (39.9804, -34.8843)
  line L288 (37.5304, -33.9843) -> (37.5304, -34.8843)
  line L289 (38.8804, -32.5343) -> (38.8804, -33.9843)
  line L290 (41.3304, -34.8843) -> (41.3304, -33.9843)
  line L291 (38.8804, -33.9843) -> (37.5304, -33.9843)
  line L292 (39.9804, -33.9843) -> (39.9804, -32.5343)
  line L293 (41.3304, -33.9843) -> (39.9804, -33.9843)
  line L294 (38.8804, -36.3343) -> (39.9804, -36.3343)
  line L295 (37.5304, -34.8843) -> (38.8804, -34.8843)
  line L296 (20.8162, -26.8093) -> (20.8162, -25.4593)
  line L297 (18.4662, -25.4593) -> (19.9162, -25.4593)
  line L298 (19.9162, -25.4593) -> (19.9162, -26.8093)
  line L299 (20.8162, -24.3593) -> (20.8162, -23.0093)
  line L300 (18.4662, -24.3593) -> (18.4662, -25.4593)
  line L301 (22.2662, -24.3593) -> (20.8162, -24.3593)
  line L302 (19.9162, -23.0093) -> (19.9162, -24.3593)
  line L303 (19.9162, -24.3593) -> (18.4662, -24.3593)
  line L304 (20.8162, -23.0093) -> (19.9162, -23.0093)
  line L305 (19.9162, -26.8093) -> (20.8162, -26.8093)
  line L306 (20.8162, -25.4593) -> (22.2662, -25.4593)
  line L307 (22.2662, -25.4593) -> (22.2662, -24.3593)
  line L308 (3.2162, -24.3593) -> (1.7662, -24.3593)
  line L309 (1.7662, -24.3593) -> (1.7662, -23.0093)
  line L310 (0.8662, -26.8093) -> (1.7662, -26.8093)
  line L311 (-0.5838, -24.3593) -> (-0.5838, -25.4593)
  line L312 (0.8662, -24.3593) -> (-0.5838, -24.3593)
  line L313 (0.8662, -25.4593) -> (0.8662, -26.8093)
  line L314 (1.7662, -23.0093) -> (0.8662, -23.0093)
  line L315 (-0.5838, -25.4593) -> (0.8662, -25.4593)
  line L316 (1.7662, -26.8093) -> (1.7662, -25.4593)
  line L317 (3.2162, -25.4593) -> (3.2162, -24.3593)
  line L318 (0.8662, -23.0093) -> (0.8662, -24.3593)
  line L319 (1.7662, -25.4593) -> (3.2162, -25.4593)
  line L320 (-14.3838, -22.3593) -> (-21.0838, -22.3593)
  line L321 (-14.3838, -27.4593) -> (-14.3838, -22.3593)
  line L322 (-21.0838, -22.3593) -> (-21.0838, -27.4593)
  line L323 (-21.0838, -27.4593) -> (-14.3838, -27.4593)
  line L324 (-18.2838, -25.5593) -> (-19.7338, -25.5593)
  line L325 (-18.2838, -24.2593) -> (-18.2838, -22.9093)
  line L326 (-17.1838, -25.5593) -> (-17.1838, -26.9093)
  line L327 (-17.1838, -26.9093) -> (-18.2838, -26.9093)
  line L328 (-15.7338, -25.5593) -> (-17.1838, -25.5593)
  line L329 (-15.7338, -24.2593) -> (-15.7338, -25.5593)
  line L330 (-19.7338, -25.5593) -> (-19.7338, -24.2593)
  line L331 (-17.1838, -24.2593) -> (-15.7338, -24.2593)
  line L332 (-19.7338, -24.2593) -> (-18.2838, -24.2593)
  line L333 (-18.2838, -22.9093) -> (-17.1838, -22.9093)
  line L334 (-18.2838, -26.9093) -> (-18.2838, -25.5593)
  line L335 (-17.1838, -22.9093) -> (-17.1838, -24.2593)
  line L336 (-24.6617, 56.5428) -> (-12.5267, 56.5428)
  line L337 (-12.5267, 56.5428) -> (-12.5267, 44.7872)
  line L338 (-12.5267, 44.7872) -> (-24.6617, 44.7872)
  line L339 (-24.6617, 44.7872) -> (-24.6617, 56.5428)
  line L340 (34.2812, 57.0639) -> (46.5476, 57.0639)
  line L341 (46.5476, 57.0639) -> (46.5476, 45.1428)
  line L342 (46.5476, 45.1428) -> (34.2812, 45.1428)
  line L343 (34.2812, 45.1428) -> (34.2812, 57.0639)
  constraint horizontal L336
  constraint vertical L337
  constraint horizontal L338
  constraint vertical L339
  constraint horizontal L340
  constraint vertical L341
  constraint horizontal L342
  constraint vertical L343